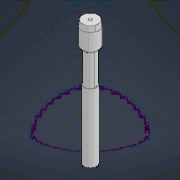
# Autodesk Inventor part: Tap
Saved by Autodesk Inventor 2025.3 (Build 293356000, 356)
## iProperties
IsCustomPart: 1
Created: 2024-06-03
Part Number: Tap
Material: Generic
Description: Dormer taps
Document SubType Name: Modeling
Designer: fablabadmin
Standard Revision: 3
Language: en-US
Size Designation: 12
Categories: <MemberInstance><Categories><Category DisplayName="CF_TAPS" InternalName="4638e9c5-4961-4352-a719-252d49e01c81" Mnemonic="CF_TAPS3"><CategoryParameter DisplayName="OAL" InternalName="031a2193-0067-493f-88ed-f98e0b7c12ca" Mnemonic="OAL"/><CategoryParameter DisplayName="TDZ" InternalName="228c7086-914f-469a-b5c9-97e5a4ae5565" Mnemonic="TDZ"/><CategoryParameter DisplayName="DCON MS" InternalName="53f33242-a9ef-47ce-b2a3-0238971920b0" Mnemonic="DCON MS"/><CategoryParameter DisplayName="LU" InternalName="807bce64-0630-47ef-b8a9-1b803567e808" Mnemonic="LU"/><CategoryParameter DisplayName="THL" InternalName="945aa789-c544-439c-8b62-7871aaaba3f5" Mnemonic="THL"/></Category><Category DisplayName="DataType" InternalName="23b78d0f-2648-40c6-8793-ca6db495c9e8" Mnemonic="DATATYPE"><CategoryParameter DisplayName="DisplayName" InternalName="05415f3d-3907-474b-a020-eb9d644f4cf3" Mnemonic="DISPLAYNAME"/><CategoryParameter DisplayName="Standard" InternalName="0c0a119c-1e12-4c84-803f-101930972f5e" Mnemonic="STANDARD"/><CategoryParameter DisplayName="Description" InternalName="13903e3d-64b1-4950-80da-f627842ea37f" Mnemonic="DESCRIPTION"/><CategoryParameter DisplayName="Designation" InternalName="2675968c-4ce5-49e0-a4f5-552d29089031" Mnemonic="DESIGNATION"/><CategoryParameter DisplayName="Default Row" InternalName="2af9ec52-faaa-4026-b378-f9fa4afca842" Mnemonic="DEFAULTROW"/><CategoryParameter DisplayName="Folder Name" InternalName="3f06958e-8713-4116-9be7-ed6184ecc97b" Mnemonic="FOLDERNAME"/><CategoryParameter DisplayName="Revision Guid" InternalName="45a75005-10b1-4dfc-8d6d-dfe629f0b93c" Mnemonic="REVISIONGUID"/><CategoryParameter DisplayName="FileName" InternalName="8b46a4cc-9585-4fed-90c3-899f57e09a73" Mnemonic="FILENAME"/><CategoryParameter DisplayName="StdsOrg" InternalName="8f5914e1-4693-403f-8ab5-d37768198c9d" Mnemonic="STDSORG"/><CategoryParameter DisplayName="Family Version" InternalName="914462f6-6e19-4b14-ba84-155b9680b1d0" Mnemonic="FAMILYREVISION"/><CategoryParameter DisplayName="Standard Revision" InternalName="91d5a463-65c2-4fde-b823-3b7fea5e8e17" Mnemonic="STANDARDREVISION"/><CategoryParameter DisplayName="Member Revision" InternalName="a65d44b9-392f-4f4f-857b-e4b3d54996fe" Mnemonic="MEMBERREVISION"/><CategoryParameter DisplayName="ClipFormat" InternalName="bc51e27b-3422-4e78-93ef-cec197ddf230" Mnemonic="CLIPFORMAT"/><CategoryParameter DisplayName="Manufacturer" InternalName="cd6c7a72-a28a-4e50-99a9-2c7f4e13e5ad" Mnemonic="MANUFACTURER"/><CategoryParameter DisplayName="InternalName" InternalName="cf1d0246-76d9-4b4a-8305-fa0409afb5c1" Mnemonic="INTERNALNAME"/><CategoryParameter DisplayName="IsMetric" InternalName="e2385c5b-1ea4-4823-96a8-8de651266ec3" Mnemonic="ISMETRIC"/><Category DisplayName="Part" InternalName="c0e0b642-3bcb-4cc8-9e80-f96d35c4afa4" Mnemonic="PART"><CategoryParameter DisplayName="Part Number" InternalName="016b6077-bfbe-49bd-92c9-d8d59c39c941" Mnemonic="PARTNUMBER"/><CategoryParameter DisplayName="Stock Number" InternalName="4dba7c1c-e26c-444e-836c-b08b433409a8" Mnemonic="STOCKNUMBER"/><CategoryParameter DisplayName="Material Key" InternalName="5c9a8adb-dd2b-4535-b97f-0a94a95fe41f" Mnemonic="MATERIALKEY"/><CategoryParameter DisplayName="Material" InternalName="818a152a-d3c3-49ca-80ee-df7d91421b8e" Mnemonic="MATERIAL"/></Category></Category></Categories><FamilyTemplate Id="Tap"><FamilyTemplateParameters><FamilyTemplateParameter ObjectType="kModelParameterObject" ValueType="xs:double" Id="12" ObjectReferenceKey="dconms"/><FamilyTemplateParameter ObjectType="kModelParameterObject" ValueType="xs:double" Id="13" ObjectReferenceKey="lu"/><FamilyTemplateParameter ObjectType="kModelParameterObject" ValueType="xs:double" Id="14" ObjectReferenceKey="oal"/><FamilyTemplateParameter ObjectType="kModelParameterObject" ValueType="xs:double" Id="15" ObjectReferenceKey="tdz"/><FamilyTemplateParameter ObjectType="kModelParameterObject" ValueType="xs:double" Id="16" ObjectReferenceKey="thl"/><FamilyTemplateParameter ObjectType="kPartComponentDefinitionObject" ValueType="xs:string" Id="27" SubObjectId="Material"/><FamilyTemplateParameter ObjectType="kPropertyObject" ValueType="xs:string" Id="29" ObjectReferenceKey="{32853F0F-3444-11d1-9E93-0060B03C1CA6}" SubObjectId="5"/><FamilyTemplateParameter ObjectType="kPropertyObject" ValueType="xs:string" Id="30" ObjectReferenceKey="{32853F0F-3444-11d1-9E93-0060B03C1CA6}" SubObjectId="52"/></FamilyTemplateParameters></FamilyTemplate><CategoryParameterMap><ParamToTemplateMap><ParamToTemplate CategoryParameter="//CategoryParameter[@InternalName='cf1d0246-76d9-4b4a-8305-fa0409afb5c1']" ConstantValue="555c8814-4a83-47ab-9e0d-220e138b2508"/><ParamToTemplate CategoryParameter="//CategoryParameter[@InternalName='45a75005-10b1-4dfc-8d6d-dfe629f0b93c']" ConstantValue="a54048ce-c516-42ea-9edf-6e60a4f9286f"/><ParamToTemplate CategoryParameter="//CategoryParameter[@InternalName='3f06958e-8713-4116-9be7-ed6184ecc97b']" ConstantValue="E002V3"/><ParamToTemplate CategoryParameter="//CategoryParameter[@InternalName='8f5914e1-4693-403f-8ab5-d37768198c9d']" TemplateParameter="21"/><ParamToTemplate CategoryParameter="//CategoryParameter[@InternalName='0c0a119c-1e12-4c84-803f-101930972f5e']" TemplateParameter="22"/><ParamToTemplate CategoryParameter="//CategoryParameter[@InternalName='91d5a463-65c2-4fde-b823-3b7fea5e8e17']" ConstantValue="3"/><ParamToTemplate CategoryParameter="//CategoryParameter[@InternalName='cd6c7a72-a28a-4e50-99a9-2c7f4e13e5ad']" TemplateParameter="24"/><ParamToTemplate CategoryParameter="//CategoryParameter[@InternalName='13903e3d-64b1-4950-80da-f627842ea37f']" ConstantValue="Dormer taps"/><ParamToTemplate CategoryParameter="//CategoryParameter[@InternalName='05415f3d-3907-474b-a020-eb9d644f4cf3']" ConstantValue="Dormer E002"/><ParamToTemplate CategoryParameter="//CategoryParameter[@InternalName='914462f6-6e19-4b14-ba84-155b9680b1d0']" ConstantValue="11"/><ParamToTemplate CategoryParameter="//CategoryParameter[@InternalName='bc51e27b-3422-4e78-93ef-cec197ddf230']" ConstantValue="CF_INVENTOR.STDPARTS"/><ParamToTemplate CategoryParameter="//CategoryParameter[@InternalName='e2385c5b-1ea4-4823-96a8-8de651266ec3']" ConstantValue="true"/><ParamToTemplate CategoryParameter="//CategoryParameter[@InternalName='2af9ec52-faaa-4026-b378-f9fa4afca842']" ConstantValue="1"/><ParamToTemplate CategoryParameter="//CategoryParameter[@InternalName='8b46a4cc-9585-4fed-90c3-899f57e09a73']" ConstantValue="E002M12"/><ParamToTemplate CategoryParameter="//CategoryParameter[@InternalName='a65d44b9-392f-4f4f-857b-e4b3d54996fe']" ConstantValue="4853e1ac-0d1d-41b5-bb01-1a8d9f2b2d17"/><ParamToTemplate CategoryParameter="//CategoryParameter[@InternalName='a65d44b9-392f-4f4f-857b-e4b3d54996fe']" ConstantValue="4853e1ac-0d1d-41b5-bb01-1a8d9f2b2d17"/><ParamToTemplate CategoryParameter="//CategoryParameter[@InternalName='2675968c-4ce5-49e0-a4f5-552d29089031']" TemplateParameter="30"/><ParamToTemplate CategoryParameter="//CategoryParameter[@InternalName='818a152a-d3c3-49ca-80ee-df7d91421b8e']" TemplateParameter="27"/><ParamToTemplate CategoryParameter="//CategoryParameter[@InternalName='016b6077-bfbe-49bd-92c9-d8d59c39c941']" TemplateParameter="29"/><ParamToTemplate CategoryParameter="//CategoryParameter[@InternalName='53f33242-a9ef-47ce-b2a3-0238971920b0']" TemplateParameter="12"/><ParamToTemplate CategoryParameter="//CategoryParameter[@InternalName='807bce64-0630-47ef-b8a9-1b803567e808']" TemplateParameter="13"/><ParamToTemplate CategoryParameter="//CategoryParameter[@InternalName='031a2193-0067-493f-88ed-f98e0b7c12ca']" TemplateParameter="14"/><ParamToTemplate CategoryParameter="//CategoryParameter[@InternalName='228c7086-914f-469a-b5c9-97e5a4ae5565']" TemplateParameter="15"/><ParamToTemplate CategoryParameter="//CategoryParameter[@InternalName='945aa789-c544-439c-8b62-7871aaaba3f5']" TemplateParameter="16"/></ParamToTemplateMap></CategoryParameterMap></MemberInstance>
Density: 1 g/cm^3
Appearance: Default
Author: fablabadmin
Autodesk Inventor part; units mm, degrees
ref_plane "YZ Plane" through (0, 0, 0) normal (1, 0, 0) x (0, 1, 0)
ref_plane "XZ Plane" through (0, 0, 0) normal (0, 1, 0) x (-1, 0, 0)
ref_plane "XY Plane" through (0, 0, 0) normal (0, 0, 1) x (1, 0, 0)
sketch "Sketch1" plane through (0, 0, 0) normal (0, 0, 1) x (1, 0, 0)
  line L0 (-7.2, 0) -> (1.2, 0) construction
  line L1 (0, -62.54) -> (0, 63.74) projected
  line L2 (0, 45.7) -> (-1.2, 44.5)
  line L3 (-1.2, 44.5) -> (-5.65, 44.5)
  line L4 (-5.65, 44.5) -> (-6, 40.5)
  line L5 (-6, 40.5) -> (-6, 28.5)
  line L6 (-4, 26.5) -> (-4, 4.5)
  line L7 (-4, 4.5) -> (-4.5, 4.5)
  line L8 (-4.5, 4.5) -> (-4.5, -44.5)
  line L9 (-4.5, -44.5) -> (0, -44.5)
  line L10 (-6, 28.5) -> (-4, 26.5)
  point P0 (0, 0)
  dimension "tdz" = 12
  dimension "d1" = 45
  dimension "d2" = 5
  dimension "thl" = 16
  dimension "lu" = 40
  dimension "oal" = 89
  dimension "d6" = 1.2
  dimension "d7" = 4
  dimension "dconms" = 9
  dimension "d9" = 8
  dimension "d11" = 45
  constraints: 18 end point, 3 perpendicular, 2 point on line, 1 horizontal, 1 vertical, 1 other
  measures "tdz" diameter of L5 L1
  measures "d1" angle of L3 L2
  measures "d2" angle of L5 L4
  measures "thl" distance from line of L5.end L3
  measures "lu" distance from line of L7.end L3
  measures "oal" distance between parallel lines of L3 L9
  measures "d6" horizontal distance of L2.end L2.start
  measures "d7" distance from line of L4.end L3
  measures "dconms" diameter of L8 L1
  measures "d9" diameter of L6 L1
  measures "d11" angle of L6 L10
revolve "Revolution1" add sketch "Sketch1" angle 360 about axis through (0, -10, 0) along (0, 1, 0)
sketch "Sketch2" plane through (0, -44.5, 0) normal (0, -1, 0) x (1, 0, 0)
  circle A0 centre (0, 0) radius 4.5 construction
  line L0 (3.55, 3.55) -> (3.55, -3.55)
  line L1 (3.55, -3.55) -> (-3.55, -3.55)
  line L2 (-3.55, -3.55) -> (-3.55, 3.55)
  line L3 (-3.55, 3.55) -> (3.55, 3.55)
  circle A1 centre (0, 0) radius 6 projected
  dimension "d12" = 7.1
  constraints: 8 end point, 1 coincident, 1 horizontal, 9 other
  measures "d12" distance of L0.start L0.end
extrude "Extrusion1" cut sketch "Sketch2" against normal blind 10
equation "\"d6\" = 0.1 * tdz"
equation "\"d7\" = 0.25 * thl"
body "Solid1"
